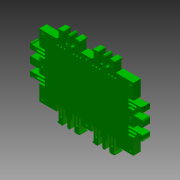
# Autodesk Inventor part: floor_base
Saved by Autodesk Inventor 2012 SP1 (Build 160190100, 190)
## iProperties
Created: 2011-10-14
Part Number: floor_base
Document SubType Name: Modeling
Designer: cramera
Density: 0.952 g/cm^3
Material: High Density Polyethylene
Mass: 189.037 g
Surface Area: 567.519 cm^2
Volume: 198.568 cm^3
Autodesk Inventor part; units mm, degrees
ref_plane "YZ Plane" through (0, 0, 0) normal (1, 0, 0) x (0, 1, 0)
ref_plane "XZ Plane" through (0, 0, 0) normal (0, 1, 0) x (-1, 0, 0)
ref_plane "XY Plane" through (0, 0, 0) normal (0, 0, 1) x (1, 0, 0)
derived "skeleton.ipt"
sketch "DRILL-THROUGH" plane through (0, 0, 0) normal (0, 0, 1) x (1, 0, 0)
  arc A0 (67.7549, 190.4821) -> (69.3424, 188.8946) centre (69.3424, 190.4821) ccw
  arc A1 (214.9174, 143.8883) -> (213.3299, 145.4758) centre (213.3299, 143.8883) ccw
  arc A2 (213.3299, 192.0696) -> (211.7424, 190.4821) centre (213.3299, 190.4821) ccw
  arc A3 (211.7424, 190.4821) -> (213.3299, 188.8946) centre (213.3299, 190.4821) ccw
  arc A4 (213.3299, 188.8946) -> (214.9174, 190.4821) centre (213.3299, 190.4821) ccw
  arc A5 (213.3299, 238.6633) -> (211.7424, 237.0758) centre (213.3299, 237.0758) ccw
  arc A6 (211.7424, 237.0758) -> (213.3299, 235.4883) centre (213.3299, 237.0758) ccw
  arc A7 (213.3299, 235.4883) -> (214.9174, 237.0758) centre (213.3299, 237.0758) ccw
  arc A8 (214.9174, 237.0758) -> (213.3299, 238.6633) centre (213.3299, 237.0758) ccw
  arc A9 (69.3424, 238.6633) -> (67.7549, 237.0758) centre (69.3424, 237.0758) ccw
  arc A10 (67.7549, 237.0758) -> (69.3424, 235.4883) centre (69.3424, 237.0758) ccw
  arc A11 (69.3424, 235.4883) -> (70.9299, 237.0758) centre (69.3424, 237.0758) ccw
  arc A12 (70.9299, 237.0758) -> (69.3424, 238.6633) centre (69.3424, 237.0758) ccw
  arc A13 (141.3362, 238.6633) -> (139.7487, 237.0758) centre (141.3362, 237.0758) ccw
  arc A14 (139.7487, 237.0758) -> (141.3362, 235.4883) centre (141.3362, 237.0758) ccw
  arc A15 (141.3362, 235.4883) -> (142.9237, 237.0758) centre (141.3362, 237.0758) ccw
  arc A16 (142.9237, 237.0758) -> (141.3362, 238.6633) centre (141.3362, 237.0758) ccw
  arc A17 (69.3424, 192.0696) -> (67.7549, 190.4821) centre (69.3424, 190.4821) ccw
  arc A18 (214.9174, 190.4821) -> (213.3299, 192.0696) centre (213.3299, 190.4821) ccw
  arc A19 (69.3424, 188.8946) -> (70.9299, 190.4821) centre (69.3424, 190.4821) ccw
  arc A20 (70.9299, 190.4821) -> (69.3424, 192.0696) centre (69.3424, 190.4821) ccw
  arc A21 (69.3424, 145.4758) -> (67.7549, 143.8883) centre (69.3424, 143.8883) ccw
  arc A22 (67.7549, 143.8883) -> (69.3424, 142.3008) centre (69.3424, 143.8883) ccw
  arc A23 (69.3424, 142.3008) -> (70.9299, 143.8883) centre (69.3424, 143.8883) ccw
  arc A24 (70.9299, 143.8883) -> (69.3424, 145.4758) centre (69.3424, 143.8883) ccw
  arc A25 (141.3362, 145.4758) -> (139.7487, 143.8883) centre (141.3362, 143.8883) ccw
  arc A26 (139.7487, 143.8883) -> (141.3362, 142.3008) centre (141.3362, 143.8883) ccw
  arc A27 (141.3362, 142.3008) -> (142.9237, 143.8883) centre (141.3362, 143.8883) ccw
  arc A28 (142.9237, 143.8883) -> (141.3362, 145.4758) centre (141.3362, 143.8883) ccw
  arc A29 (213.3299, 145.4758) -> (211.7424, 143.8883) centre (213.3299, 143.8883) ccw
  arc A30 (211.7424, 143.8883) -> (213.3299, 142.3008) centre (213.3299, 143.8883) ccw
  arc A31 (213.3299, 142.3008) -> (214.9174, 143.8883) centre (213.3299, 143.8883) ccw
  constraints: 64 point on circle, 32 centre point
sketch "STOCK_12MM" plane through (0, 0, 0) normal (0, 0, 1) x (1, 0, 0)
  line L0 (0, 0) -> (457.2, 0)
  line L1 (457.2, 0) -> (457.2, 914.4)
  line L2 (457.2, 914.4) -> (0, 914.4)
  line L3 (0, 914.4) -> (0, 0)
  line L4 (457.2, 914.4) -> (457.2, 0)
  constraints: 10 end point
sketch "THROUGH-CUT" plane through (0, 0, 0) normal (0, 0, 1) x (1, 0, 0)
  arc A0 (155.4332, 135.2959) -> (157.0207, 133.7099) centre (157.0207, 135.2974) ccw
  line L0 (155.4332, 135.2959) -> (155.4332, 146.8258)
  arc A1 (157.0207, 148.4133) -> (155.4332, 146.8258) centre (157.0207, 146.8258) ccw
  line L1 (157.0207, 148.4133) -> (157.1477, 148.4133)
  arc A2 (158.7352, 146.8258) -> (157.1477, 148.4133) centre (157.1477, 146.8258) ccw
  line L2 (158.7352, 146.8258) -> (158.7352, 135.2974)
  arc A3 (157.1477, 133.7099) -> (158.7352, 135.2974) centre (157.1477, 135.2974) ccw
  line L3 (157.1477, 133.7099) -> (157.0207, 133.7099)
  arc A4 (208.8049, 209.5956) -> (210.3924, 208.0081) centre (210.3924, 209.5956) ccw
  line L4 (210.3924, 208.0081) -> (221.9209, 208.0081)
  arc A5 (221.9209, 208.0081) -> (223.5084, 209.5956) centre (221.9209, 209.5956) ccw
  line L5 (223.5084, 209.5956) -> (223.5084, 209.7226)
  arc A6 (223.5084, 209.7226) -> (221.9209, 211.3101) centre (221.9209, 209.7226) ccw
  line L6 (221.9209, 211.3101) -> (210.3924, 211.3101)
  arc A7 (210.3924, 211.3101) -> (208.8049, 209.7226) centre (210.3924, 209.7226) ccw
  line L7 (208.8049, 209.7226) -> (208.8049, 209.5956)
  arc A8 (181.0872, 135.2974) -> (182.6747, 133.7099) centre (182.6747, 135.2974) ccw
  line L8 (182.6747, 133.7099) -> (182.8017, 133.7099)
  arc A9 (182.8017, 133.7099) -> (184.3892, 135.2974) centre (182.8017, 135.2974) ccw
  line L9 (184.3892, 135.2974) -> (184.3892, 146.8258)
  arc A10 (184.3892, 146.8258) -> (182.8017, 148.4133) centre (182.8017, 146.8258) ccw
  line L10 (182.8017, 148.4133) -> (182.6747, 148.4133)
  arc A11 (182.6747, 148.4133) -> (181.0872, 146.8258) centre (182.6747, 146.8258) ccw
  line L11 (181.0872, 146.8258) -> (181.0872, 135.2974)
  arc A12 (123.9372, 135.2974) -> (125.5247, 133.7099) centre (125.5247, 135.2974) ccw
  line L12 (125.5247, 133.7099) -> (125.6517, 133.7099)
  arc A13 (125.6517, 133.7099) -> (127.2392, 135.2974) centre (125.6517, 135.2974) ccw
  line L13 (127.2392, 135.2974) -> (127.2392, 146.8258)
  arc A14 (127.2392, 146.8258) -> (125.6517, 148.4133) centre (125.6517, 146.8258) ccw
  line L14 (125.6517, 148.4133) -> (125.5247, 148.4133)
  arc A15 (125.5247, 148.4133) -> (123.9372, 146.8258) centre (125.5247, 146.8258) ccw
  line L15 (123.9372, 146.8258) -> (123.9372, 135.2974)
  arc A16 (98.2832, 135.2974) -> (99.8707, 133.7099) centre (99.8707, 135.2974) ccw
  line L16 (98.2832, 135.2974) -> (98.2832, 146.8258)
  arc A17 (99.8707, 148.4133) -> (98.2832, 146.8258) centre (99.8707, 146.8258) ccw
  line L17 (99.8707, 148.4133) -> (99.9977, 148.4133)
  arc A18 (101.5852, 146.8258) -> (99.9977, 148.4133) centre (99.9977, 146.8258) ccw
  line L18 (101.5852, 146.8258) -> (101.5852, 135.2974)
  arc A19 (99.9977, 133.7099) -> (101.5852, 135.2974) centre (99.9977, 135.2974) ccw
  line L19 (99.9977, 133.7099) -> (99.8707, 133.7099)
  arc A20 (181.0872, 234.1383) -> (182.6747, 232.5508) centre (182.6747, 234.1383) ccw
  line L20 (181.0872, 234.1383) -> (181.0872, 245.6668)
  arc A21 (182.6747, 247.2543) -> (181.0872, 245.6668) centre (182.6747, 245.6668) ccw
  line L21 (182.6747, 247.2543) -> (182.8017, 247.2543)
  arc A22 (184.3892, 245.6668) -> (182.8017, 247.2543) centre (182.8017, 245.6668) ccw
  line L22 (184.3892, 245.6668) -> (184.3892, 234.1383)
  arc A23 (182.8017, 232.5508) -> (184.3892, 234.1383) centre (182.8017, 234.1383) ccw
  line L23 (182.8017, 232.5508) -> (182.6747, 232.5508)
  arc A24 (73.8674, 209.7226) -> (72.2799, 211.3101) centre (72.2799, 209.7226) ccw
  line L24 (73.8674, 209.7226) -> (73.8674, 209.5956)
  arc A25 (72.2799, 208.0081) -> (73.8674, 209.5956) centre (72.2799, 209.5956) ccw
  line L25 (72.2799, 208.0081) -> (60.7515, 208.0081)
  arc A26 (59.164, 209.5956) -> (60.7515, 208.0081) centre (60.7515, 209.5956) ccw
  line L26 (59.164, 209.5956) -> (59.164, 209.7226)
  arc A27 (60.7515, 211.3101) -> (59.164, 209.7226) centre (60.7515, 209.7226) ccw
  line L27 (60.7515, 211.3101) -> (72.2799, 211.3101)
  arc A28 (73.8674, 171.3686) -> (72.2799, 172.9561) centre (72.2799, 171.3686) ccw
  line L28 (72.2799, 172.9561) -> (60.7515, 172.9561)
  arc A29 (60.7515, 172.9561) -> (59.164, 171.3686) centre (60.7515, 171.3686) ccw
  line L29 (59.164, 171.3686) -> (59.164, 171.2416)
  arc A30 (59.164, 171.2416) -> (60.7515, 169.6541) centre (60.7515, 171.2416) ccw
  line L30 (60.7515, 169.6541) -> (72.2799, 169.6541)
  arc A31 (72.2799, 169.6541) -> (73.8674, 171.2416) centre (72.2799, 171.2416) ccw
  line L31 (73.8674, 171.2416) -> (73.8674, 171.3686)
  arc A32 (123.9372, 234.1383) -> (125.5247, 232.5508) centre (125.5247, 234.1383) ccw
  line L32 (123.9372, 234.1383) -> (123.9372, 245.6668)
  arc A33 (125.5247, 247.2543) -> (123.9372, 245.6668) centre (125.5247, 245.6668) ccw
  line L33 (125.5247, 247.2543) -> (125.6517, 247.2543)
  arc A34 (127.2392, 245.6668) -> (125.6517, 247.2543) centre (125.6517, 245.6668) ccw
  line L34 (127.2392, 245.6668) -> (127.2392, 234.1383)
  arc A35 (125.6517, 232.5508) -> (127.2392, 234.1383) centre (125.6517, 234.1383) ccw
  line L35 (125.6517, 232.5508) -> (125.5247, 232.5508)
  arc A36 (223.5084, 171.3686) -> (221.9209, 172.9561) centre (221.9209, 171.3686) ccw
  line L36 (223.5084, 171.3686) -> (223.5084, 171.2416)
  arc A37 (221.9209, 169.6541) -> (223.5084, 171.2416) centre (221.9209, 171.2416) ccw
  line L37 (221.9209, 169.6541) -> (210.3924, 169.6541)
  arc A38 (208.8049, 171.2416) -> (210.3924, 169.6541) centre (210.3924, 171.2416) ccw
  line L38 (208.8049, 171.2416) -> (208.8049, 171.3686)
  arc A39 (210.3924, 172.9561) -> (208.8049, 171.3686) centre (210.3924, 171.3686) ccw
  line L39 (210.3924, 172.9561) -> (221.9209, 172.9561)
  arc A40 (155.4332, 234.1383) -> (157.0207, 232.5508) centre (157.0207, 234.1383) ccw
  line L40 (157.0207, 232.5508) -> (157.1477, 232.5508)
  arc A41 (157.1477, 232.5508) -> (158.7352, 234.1383) centre (157.1477, 234.1383) ccw
  line L41 (158.7352, 234.1383) -> (158.7352, 245.6668)
  arc A42 (158.7352, 245.6668) -> (157.1477, 247.2543) centre (157.1477, 245.6668) ccw
  line L42 (157.1477, 247.2543) -> (157.0207, 247.2543)
  arc A43 (157.0207, 247.2543) -> (155.4332, 245.6668) centre (157.0207, 245.6668) ccw
  line L43 (155.4332, 245.6668) -> (155.4332, 234.1383)
  arc A44 (99.8707, 247.2543) -> (98.2832, 245.6668) centre (99.8707, 245.6668) ccw
  line L44 (98.2832, 245.6668) -> (98.2832, 234.1383)
  arc A45 (98.2832, 234.1383) -> (99.8707, 232.5508) centre (99.8707, 234.1383) ccw
  line L45 (99.8707, 232.5508) -> (99.9977, 232.5508)
  arc A46 (99.9977, 232.5508) -> (101.5852, 234.1383) centre (99.9977, 234.1383) ccw
  line L46 (101.5852, 234.1383) -> (101.5852, 245.6668)
  arc A47 (101.5852, 245.6668) -> (99.9977, 247.2543) centre (99.9977, 245.6668) ccw
  line L47 (99.9977, 247.2543) -> (99.8707, 247.2543)
  line L48 (102.0297, 123.6483) -> (98.3268, 123.6483)
  line L49 (98.3268, 123.6483) -> (94.7272, 124.4704)
  line L50 (94.7272, 124.4704) -> (94.7272, 126.1883)
  line L51 (94.7272, 126.1883) -> (96.2512, 127.4583)
  line L52 (96.2512, 127.4583) -> (96.2512, 130.0856)
  line L53 (96.2512, 130.0856) -> (96.2512, 146.8258)
  arc A48 (96.2512, 146.8258) -> (94.6637, 148.4133) centre (94.6637, 146.8258) ccw
  line L54 (94.6637, 148.4133) -> (94.5367, 148.4133)
  arc A49 (94.5367, 148.4133) -> (92.9492, 146.8258) centre (94.5367, 146.8258) ccw
  line L55 (92.9492, 146.8258) -> (92.9492, 138.8883)
  line L56 (92.9492, 138.8883) -> (64.3424, 138.8883)
  line L57 (64.3424, 138.8883) -> (64.3424, 164.3201)
  line L58 (64.3424, 164.3201) -> (72.2799, 164.3201)
  arc A50 (72.2799, 164.3201) -> (73.8674, 165.9076) centre (72.2799, 165.9076) ccw
  line L59 (73.8674, 165.9076) -> (73.8674, 166.0346)
  arc A51 (73.8674, 166.0346) -> (72.2799, 167.6221) centre (72.2799, 166.0346) ccw
  line L60 (72.2799, 167.6221) -> (55.5397, 167.6221)
  line L61 (55.5397, 167.6221) -> (52.9124, 167.6221)
  line L62 (52.9124, 167.6221) -> (51.6424, 166.0981)
  line L63 (51.6424, 166.0981) -> (49.9245, 166.0981)
  line L64 (49.9245, 166.0981) -> (49.1024, 169.6976)
  line L65 (49.1024, 169.6976) -> (49.1024, 173.4027)
  arc A52 (50.6899, 174.9881) -> (49.1024, 173.4027) centre (50.6899, 173.4006) ccw
  line L66 (50.6899, 174.9881) -> (72.2799, 174.9881)
  arc A53 (72.2799, 174.9881) -> (73.8674, 176.5756) centre (72.2799, 176.5756) ccw
  line L67 (73.8674, 176.5756) -> (73.8674, 176.7026)
  arc A54 (73.8674, 176.7026) -> (72.2799, 178.2901) centre (72.2799, 176.7026) ccw
  line L68 (72.2799, 178.2901) -> (64.3424, 178.2901)
  line L69 (64.3424, 178.2901) -> (64.3424, 182.522)
  arc A55 (64.3424, 182.522) -> (62.0974, 184.7671) centre (63.2199, 183.6445) ccw
  line L70 (62.0974, 184.7671) -> (50.6899, 184.7671)
  line L71 (50.6899, 184.7671) -> (49.1024, 186.3546)
  line L72 (49.1024, 186.3546) -> (49.1024, 194.6096)
  line L73 (49.1024, 194.6096) -> (50.6899, 196.1971)
  line L74 (50.6899, 196.1971) -> (62.0974, 196.1971)
  arc A56 (62.0974, 196.1971) -> (64.3424, 198.4421) centre (63.2199, 197.3196) ccw
  line L75 (64.3424, 198.4421) -> (64.3424, 202.6741)
  line L76 (64.3424, 202.6741) -> (72.2799, 202.6741)
  arc A57 (72.2799, 202.6741) -> (73.8674, 204.2616) centre (72.2799, 204.2616) ccw
  line L77 (73.8674, 204.2616) -> (73.8674, 204.3886)
  arc A58 (73.8674, 204.3886) -> (72.2799, 205.9761) centre (72.2799, 204.3886) ccw
  line L78 (72.2799, 205.9761) -> (50.6899, 205.9761)
  arc A59 (49.1024, 207.5636) -> (50.6899, 205.9761) centre (50.6899, 207.5636) ccw
  line L79 (49.1024, 207.5636) -> (49.1024, 211.2665)
  line L80 (49.1024, 211.2665) -> (49.9245, 214.8661)
  line L81 (49.9245, 214.8661) -> (51.6424, 214.8661)
  line L82 (51.6424, 214.8661) -> (52.9124, 213.3421)
  line L83 (52.9124, 213.3421) -> (55.5397, 213.3421)
  line L84 (55.5397, 213.3421) -> (72.2799, 213.3421)
  arc A60 (72.2799, 213.3421) -> (73.8674, 214.9296) centre (72.2799, 214.9296) ccw
  line L85 (73.8674, 214.9296) -> (73.8674, 215.0566)
  arc A61 (73.8674, 215.0566) -> (72.2799, 216.6441) centre (72.2799, 215.0566) ccw
  line L86 (72.2799, 216.6441) -> (64.3424, 216.6441)
  line L87 (64.3424, 216.6441) -> (64.3424, 242.0758)
  line L88 (64.3424, 242.0758) -> (92.9492, 242.0758)
  line L89 (92.9492, 242.0758) -> (92.9492, 234.1383)
  arc A62 (92.9492, 234.1383) -> (94.5367, 232.5508) centre (94.5367, 234.1383) ccw
  line L90 (94.5367, 232.5508) -> (94.6637, 232.5508)
  arc A63 (94.6637, 232.5508) -> (96.2512, 234.1383) centre (94.6637, 234.1383) ccw
  line L91 (96.2512, 234.1383) -> (96.2512, 250.8785)
  line L92 (96.2512, 250.8785) -> (96.2512, 253.5058)
  line L93 (96.2512, 253.5058) -> (94.7272, 254.7758)
  line L94 (94.7272, 254.7758) -> (94.7272, 256.4937)
  line L95 (94.7272, 256.4937) -> (98.3268, 257.3158)
  line L96 (98.3268, 257.3158) -> (102.0297, 257.3158)
  arc A64 (103.6172, 255.7283) -> (102.0297, 257.3158) centre (102.0297, 255.7283) ccw
  line L97 (103.6172, 255.7283) -> (103.6172, 234.1383)
  arc A65 (103.6172, 234.1383) -> (105.2047, 232.5508) centre (105.2047, 234.1383) ccw
  line L98 (105.2047, 232.5508) -> (105.3317, 232.5508)
  arc A66 (105.3317, 232.5508) -> (106.9192, 234.1383) centre (105.3317, 234.1383) ccw
  line L99 (106.9192, 234.1383) -> (106.9192, 242.0758)
  line L100 (106.9192, 242.0758) -> (107.9761, 242.0758)
  arc A67 (107.9761, 242.0758) -> (110.2212, 244.3209) centre (109.0987, 243.1984) ccw
  line L101 (110.2212, 244.3209) -> (110.2212, 255.7283)
  line L102 (110.2212, 255.7283) -> (111.8087, 257.3158)
  line L103 (111.8087, 257.3158) -> (113.7137, 257.3158)
  line L104 (113.7137, 257.3158) -> (115.3012, 255.7283)
  line L105 (115.3012, 255.7283) -> (115.3012, 244.3209)
  arc A68 (115.3012, 244.3209) -> (117.5463, 242.0758) centre (116.4237, 243.1984) ccw
  line L106 (117.5463, 242.0758) -> (118.6032, 242.0758)
  line L107 (118.6032, 242.0758) -> (118.6032, 234.1383)
  arc A69 (118.6032, 234.1383) -> (120.1907, 232.5508) centre (120.1907, 234.1383) ccw
  line L108 (120.1907, 232.5508) -> (120.3177, 232.5508)
  arc A70 (120.3177, 232.5508) -> (121.9052, 234.1383) centre (120.3177, 234.1383) ccw
  line L109 (121.9052, 234.1383) -> (121.9052, 255.7283)
  arc A71 (123.4905, 257.3158) -> (121.9052, 255.7283) centre (123.4927, 255.7283) ccw
  line L110 (123.4905, 257.3158) -> (127.1956, 257.3158)
  line L111 (127.1956, 257.3158) -> (130.7952, 256.4937)
  line L112 (130.7952, 256.4937) -> (130.7952, 254.7758)
  line L113 (130.7952, 254.7758) -> (129.2712, 253.5058)
  line L114 (129.2712, 253.5058) -> (129.2712, 250.8785)
  line L115 (129.2712, 250.8785) -> (129.2712, 234.1383)
  arc A72 (129.2712, 234.1383) -> (130.8587, 232.5508) centre (130.8587, 234.1383) ccw
  line L116 (130.8587, 232.5508) -> (130.9857, 232.5508)
  arc A73 (130.9857, 232.5508) -> (132.5732, 234.1383) centre (130.9857, 234.1383) ccw
  line L117 (132.5732, 234.1383) -> (132.5732, 242.0758)
  line L118 (132.5732, 242.0758) -> (150.0992, 242.0758)
  line L119 (150.0992, 242.0758) -> (150.0992, 234.1383)
  arc A74 (150.0992, 234.1383) -> (151.6867, 232.5508) centre (151.6867, 234.1383) ccw
  line L120 (151.6867, 232.5508) -> (151.8137, 232.5508)
  arc A75 (151.8137, 232.5508) -> (153.4012, 234.1383) centre (151.8137, 234.1383) ccw
  line L121 (153.4012, 234.1383) -> (153.4012, 250.8785)
  line L122 (153.4012, 250.8785) -> (153.4012, 253.5058)
  line L123 (153.4012, 253.5058) -> (151.8772, 254.7758)
  line L124 (151.8772, 254.7758) -> (151.8772, 256.4937)
  line L125 (151.8772, 256.4937) -> (155.4768, 257.3158)
  line L126 (155.4768, 257.3158) -> (159.1819, 257.3158)
  arc A76 (160.7672, 255.7283) -> (159.1819, 257.3158) centre (159.1797, 255.7283) ccw
  line L127 (160.7672, 255.7283) -> (160.7672, 234.1383)
  arc A77 (160.7672, 234.1383) -> (162.3547, 232.5508) centre (162.3547, 234.1383) ccw
  line L128 (162.3547, 232.5508) -> (162.4817, 232.5508)
  arc A78 (162.4817, 232.5508) -> (164.0692, 234.1383) centre (162.4817, 234.1383) ccw
  line L129 (164.0692, 234.1383) -> (164.0692, 242.0758)
  line L130 (164.0692, 242.0758) -> (165.1261, 242.0758)
  arc A79 (165.1261, 242.0758) -> (167.3712, 244.3209) centre (166.2487, 243.1984) ccw
  line L131 (167.3712, 244.3209) -> (167.3712, 255.7283)
  line L132 (167.3712, 255.7283) -> (168.9587, 257.3158)
  line L133 (168.9587, 257.3158) -> (170.8637, 257.3158)
  line L134 (170.8637, 257.3158) -> (172.4512, 255.7283)
  line L135 (172.4512, 255.7283) -> (172.4512, 244.3209)
  arc A80 (172.4512, 244.3209) -> (174.6963, 242.0758) centre (173.5737, 243.1984) ccw
  line L136 (174.6963, 242.0758) -> (175.7532, 242.0758)
  line L137 (175.7532, 242.0758) -> (175.7532, 234.1383)
  arc A81 (175.7532, 234.1383) -> (177.3407, 232.5508) centre (177.3407, 234.1383) ccw
  line L138 (177.3407, 232.5508) -> (177.4677, 232.5508)
  arc A82 (177.4677, 232.5508) -> (179.0552, 234.1383) centre (177.4677, 234.1383) ccw
  line L139 (179.0552, 234.1383) -> (179.0552, 255.7283)
  arc A83 (180.6427, 257.3158) -> (179.0552, 255.7283) centre (180.6427, 255.7283) ccw
  line L140 (180.6427, 257.3158) -> (184.3456, 257.3158)
  line L141 (184.3456, 257.3158) -> (187.9452, 256.4937)
  line L142 (187.9452, 256.4937) -> (187.9452, 254.7758)
  line L143 (187.9452, 254.7758) -> (186.4212, 253.5058)
  line L144 (186.4212, 253.5058) -> (186.4212, 250.8785)
  line L145 (186.4212, 250.8785) -> (186.4212, 234.1383)
  arc A84 (186.4212, 234.1383) -> (188.0087, 232.5508) centre (188.0087, 234.1383) ccw
  line L146 (188.0087, 232.5508) -> (188.1357, 232.5508)
  arc A85 (188.1357, 232.5508) -> (189.7232, 234.1383) centre (188.1357, 234.1383) ccw
  line L147 (189.7232, 234.1383) -> (189.7232, 242.0758)
  line L148 (189.7232, 242.0758) -> (218.3299, 242.0758)
  line L149 (218.3299, 242.0758) -> (218.3299, 216.6441)
  line L150 (218.3299, 216.6441) -> (210.3924, 216.6441)
  arc A86 (210.3924, 216.6441) -> (208.8049, 215.0566) centre (210.3924, 215.0566) ccw
  line L151 (208.8049, 215.0566) -> (208.8049, 214.9296)
  arc A87 (208.8049, 214.9296) -> (210.3924, 213.3421) centre (210.3924, 214.9296) ccw
  line L152 (210.3924, 213.3421) -> (227.1327, 213.3421)
  line L153 (227.1327, 213.3421) -> (229.7599, 213.3421)
  line L154 (229.7599, 213.3421) -> (231.0299, 214.8661)
  line L155 (231.0299, 214.8661) -> (232.7479, 214.8661)
  line L156 (232.7479, 214.8661) -> (233.5699, 211.2665)
  line L157 (233.5699, 211.2665) -> (233.5699, 207.5636)
  arc A88 (231.9824, 205.9761) -> (233.5699, 207.5636) centre (231.9824, 207.5636) ccw
  line L158 (231.9824, 205.9761) -> (210.3924, 205.9761)
  arc A89 (210.3924, 205.9761) -> (208.8049, 204.3886) centre (210.3924, 204.3886) ccw
  line L159 (208.8049, 204.3886) -> (208.8049, 204.2616)
  arc A90 (208.8049, 204.2616) -> (210.3924, 202.6741) centre (210.3924, 204.2616) ccw
  line L160 (210.3924, 202.6741) -> (218.3299, 202.6741)
  line L161 (218.3299, 202.6741) -> (218.3299, 198.4421)
  arc A91 (218.3299, 198.4421) -> (220.575, 196.1971) centre (219.4525, 197.3196) ccw
  line L162 (220.575, 196.1971) -> (231.9824, 196.1971)
  line L163 (231.9824, 196.1971) -> (233.5699, 194.6096)
  line L164 (233.5699, 194.6096) -> (233.5699, 186.3546)
  line L165 (233.5699, 186.3546) -> (231.9824, 184.7671)
  line L166 (231.9824, 184.7671) -> (220.575, 184.7671)
  arc A92 (220.575, 184.7671) -> (218.3299, 182.522) centre (219.4525, 183.6445) ccw
  line L167 (218.3299, 182.522) -> (218.3299, 178.2901)
  line L168 (218.3299, 178.2901) -> (210.3924, 178.2901)
  arc A93 (210.3924, 178.2901) -> (208.8049, 176.7026) centre (210.3924, 176.7026) ccw
  line L169 (208.8049, 176.7026) -> (208.8049, 176.5756)
  arc A94 (208.8049, 176.5756) -> (210.3924, 174.9881) centre (210.3924, 176.5756) ccw
  line L170 (210.3924, 174.9881) -> (231.9824, 174.9881)
  arc A95 (233.5699, 173.4027) -> (231.9824, 174.9881) centre (231.9824, 173.4006) ccw
  line L171 (233.5699, 173.4027) -> (233.5699, 169.6976)
  line L172 (233.5699, 169.6976) -> (232.7479, 166.0981)
  line L173 (232.7479, 166.0981) -> (231.0299, 166.0981)
  line L174 (231.0299, 166.0981) -> (229.7599, 167.6221)
  line L175 (229.7599, 167.6221) -> (227.1327, 167.6221)
  line L176 (227.1327, 167.6221) -> (210.3924, 167.6221)
  arc A96 (210.3924, 167.6221) -> (208.8049, 166.0346) centre (210.3924, 166.0346) ccw
  line L177 (208.8049, 166.0346) -> (208.8049, 165.9076)
  arc A97 (208.8049, 165.9076) -> (210.3924, 164.3201) centre (210.3924, 165.9076) ccw
  line L178 (210.3924, 164.3201) -> (218.3299, 164.3201)
  line L179 (218.3299, 164.3201) -> (218.3299, 138.8883)
  line L180 (218.3299, 138.8883) -> (189.7232, 138.8883)
  line L181 (189.7232, 138.8883) -> (189.7232, 146.8258)
  arc A98 (189.7232, 146.8258) -> (188.1357, 148.4133) centre (188.1357, 146.8258) ccw
  line L182 (188.1357, 148.4133) -> (188.0087, 148.4133)
  arc A99 (188.0087, 148.4133) -> (186.4212, 146.8258) centre (188.0087, 146.8258) ccw
  line L183 (186.4212, 146.8258) -> (186.4212, 130.0856)
  line L184 (186.4212, 130.0856) -> (186.4212, 127.4583)
  line L185 (186.4212, 127.4583) -> (187.9452, 126.1883)
  line L186 (187.9452, 126.1883) -> (187.9452, 124.4704)
  line L187 (187.9452, 124.4704) -> (184.3456, 123.6483)
  line L188 (184.3456, 123.6483) -> (180.6427, 123.6483)
  arc A100 (179.0552, 125.2358) -> (180.6427, 123.6483) centre (180.6427, 125.2358) ccw
  line L189 (179.0552, 125.2358) -> (179.0552, 146.8258)
  arc A101 (179.0552, 146.8258) -> (177.4677, 148.4133) centre (177.4677, 146.8258) ccw
  line L190 (177.4677, 148.4133) -> (177.3407, 148.4133)
  arc A102 (177.3407, 148.4133) -> (175.7532, 146.8258) centre (177.3407, 146.8258) ccw
  line L191 (175.7532, 146.8258) -> (175.7532, 138.8883)
  line L192 (175.7532, 138.8883) -> (174.6963, 138.8883)
  arc A103 (174.6963, 138.8883) -> (172.4512, 136.6433) centre (173.5737, 137.7658) ccw
  line L193 (172.4512, 136.6433) -> (172.4512, 125.2358)
  line L194 (172.4512, 125.2358) -> (170.8637, 123.6483)
  line L195 (170.8637, 123.6483) -> (168.9587, 123.6483)
  line L196 (168.9587, 123.6483) -> (167.3712, 125.2358)
  line L197 (167.3712, 125.2358) -> (167.3712, 136.6433)
  arc A104 (167.3712, 136.6433) -> (165.1261, 138.8883) centre (166.2487, 137.7658) ccw
  line L198 (165.1261, 138.8883) -> (164.0692, 138.8883)
  line L199 (164.0692, 138.8883) -> (164.0692, 146.8258)
  arc A105 (164.0692, 146.8258) -> (162.4817, 148.4133) centre (162.4817, 146.8258) ccw
  line L200 (162.4817, 148.4133) -> (162.3547, 148.4133)
  arc A106 (162.3547, 148.4133) -> (160.7672, 146.8258) centre (162.3547, 146.8258) ccw
  line L201 (160.7672, 146.8258) -> (160.7672, 125.2358)
  arc A107 (159.1819, 123.6483) -> (160.7672, 125.2358) centre (159.1797, 125.2358) ccw
  line L202 (159.1819, 123.6483) -> (155.4768, 123.6483)
  line L203 (155.4768, 123.6483) -> (151.8772, 124.4704)
  line L204 (151.8772, 124.4704) -> (151.8772, 126.1883)
  line L205 (151.8772, 126.1883) -> (153.4012, 127.4583)
  line L206 (153.4012, 127.4583) -> (153.4012, 130.0856)
  line L207 (153.4012, 130.0856) -> (153.4012, 146.8258)
  arc A108 (153.4012, 146.8258) -> (151.8137, 148.4133) centre (151.8137, 146.8258) ccw
  line L208 (151.8137, 148.4133) -> (151.6867, 148.4133)
  arc A109 (151.6867, 148.4133) -> (150.0992, 146.8258) centre (151.6867, 146.8258) ccw
  line L209 (150.0992, 146.8258) -> (150.0992, 138.8883)
  line L210 (150.0992, 138.8883) -> (132.5732, 138.8883)
  line L211 (132.5732, 138.8883) -> (132.5732, 146.8258)
  arc A110 (132.5732, 146.8258) -> (130.9857, 148.4133) centre (130.9857, 146.8258) ccw
  line L212 (130.9857, 148.4133) -> (130.8587, 148.4133)
  arc A111 (130.8587, 148.4133) -> (129.2712, 146.8258) centre (130.8587, 146.8258) ccw
  line L213 (129.2712, 146.8258) -> (129.2712, 130.0856)
  line L214 (129.2712, 130.0856) -> (129.2712, 127.4583)
  line L215 (129.2712, 127.4583) -> (130.7952, 126.1883)
  line L216 (130.7952, 126.1883) -> (130.7952, 124.4704)
  line L217 (130.7952, 124.4704) -> (127.1956, 123.6483)
  line L218 (127.1956, 123.6483) -> (123.4905, 123.6483)
  arc A112 (121.9052, 125.2358) -> (123.4905, 123.6483) centre (123.4927, 125.2358) ccw
  line L219 (121.9052, 125.2358) -> (121.9052, 146.8258)
  arc A113 (121.9052, 146.8258) -> (120.3177, 148.4133) centre (120.3177, 146.8258) ccw
  line L220 (120.3177, 148.4133) -> (120.1907, 148.4133)
  arc A114 (120.1907, 148.4133) -> (118.6032, 146.8258) centre (120.1907, 146.8258) ccw
  line L221 (118.6032, 146.8258) -> (118.6032, 138.8883)
  line L222 (118.6032, 138.8883) -> (117.5463, 138.8883)
  arc A115 (117.5463, 138.8883) -> (115.3012, 136.6433) centre (116.4237, 137.7658) ccw
  line L223 (115.3012, 136.6433) -> (115.3012, 125.2358)
  line L224 (115.3012, 125.2358) -> (113.7137, 123.6483)
  line L225 (113.7137, 123.6483) -> (111.8087, 123.6483)
  line L226 (111.8087, 123.6483) -> (110.2212, 125.2358)
  line L227 (110.2212, 125.2358) -> (110.2212, 136.6433)
  arc A116 (110.2212, 136.6433) -> (107.9761, 138.8883) centre (109.0987, 137.7658) ccw
  line L228 (107.9761, 138.8883) -> (106.9192, 138.8883)
  line L229 (106.9192, 138.8883) -> (106.9192, 146.8258)
  arc A117 (106.9192, 146.8258) -> (105.3317, 148.4133) centre (105.3317, 146.8258) ccw
  line L230 (105.3317, 148.4133) -> (105.2047, 148.4133)
  arc A118 (105.2047, 148.4133) -> (103.6172, 146.8258) centre (105.2047, 146.8258) ccw
  line L231 (103.6172, 146.8258) -> (103.6172, 125.2358)
  arc A119 (102.0297, 123.6483) -> (103.6172, 125.2358) centre (102.0297, 125.2358) ccw
  constraints: 464 end point, 240 point on circle, 120 centre point
extrude "Extrusion1" add sketch "THROUGH-CUT" along normal blind 12
extrude "Extrusion2" cut sketch "DRILL-THROUGH" along normal through all
equation "\"d1\" = StockThickness"
equation "\"StockThickness\" = 12"
body "Solid1"
